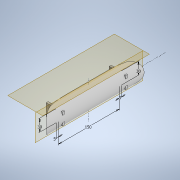
# Autodesk Inventor part: Deckel_Parachute_4
Saved by Autodesk Inventor 2020 (Build 240168000, 168)
## iProperties
Created: 2022-01-25
Part Number: Deckel_Parachute_4
Material: Generisch
Document SubType Name: Modeling
Designer: sp
Density: 1 g/cm^3
Appearance: Vorgabe
Author: sp
## iProperties of the stored document _3D-Druck.ipt
Created: 2022-05-02
Part Number: _3D-Druck
Material: Generisch
Document SubType Name: Modeling
Designer: sp
Density: 1 g/cm^3
Appearance: Vorgabe
Author: sp
Autodesk Inventor part; units mm, degrees
ref_plane "XY Plane" through (0, 0, 0) normal (0, 0, 1) x (1, 0, 0)
sketch "Skizze1" plane through (0, 0, 0) normal (0, 0, 1) x (1, 0, 0)
  circle A0 centre (0, 0) radius 31
  circle A1 centre (0, 0) radius 29
  dimension "d0" = 62
  dimension "d1" = 58
  constraints: 2 centre point, 2 coincident
  measures "d0" diameter of A0
  measures "d1" diameter of A1
extrude "Extrusion1" add sketch "Skizze1" along normal mid plane 300
sketch "Skizze2" plane through (0, 0, 0) normal (0, 1, 0) x (-1, 0, 0)
  line L0 (-11, 169.5773) -> (-11, -169.8146) construction
  line L1 (-74.8376, 0) -> (82.6362, 0) construction
  line L2 (-11, 75) -> (-11, -75)
  line L3 (-31, -150) -> (-31, 150) projected
  line L4 (31, 150) -> (-31, 150) projected
  line L5 (-31, -150) -> (31, -150) projected
  spline S0 degree 2 poles (-11, 75) (-17.8298, 136.4739) (-72.8449, 128.3193) knots 0 0 0 1 1 1
  spline S1 degree 2 poles (-11, -75) (-17.6171, -136.2673) (-74.8376, -130) knots 0 0 0 1 1 1
  line L6 (-72.8449, 128.3193) -> (-74.8376, -130)
  line L7 (-31, 120) -> (-31, 150)
  line L8 (-31, 150) -> (31, 150)
  line L9 (31, 150) -> (31, -150)
  line L10 (31, -150) -> (31, 150) projected
  line L11 (31, -150) -> (-31, -150)
  line L12 (-31, -150) -> (-31, -120)
  point P0 (0, 0)
  dimension "d4" = 11
  dimension "d5" = 150
  dimension "d6" = 30
  dimension "d7" = 30
  constraints: 18 end point, 5 point on line, 3 perpendicular, 2 collinear, 1 horizontal, 1 symmetric about line, 1 vertical, 6 other
  measures "d4" distance from line of point (0, 0) L0
  measures "d5" distance of L2.start L2.end
  measures "d6" distance from line of L7.start L4
  measures "d7" distance from line of L12.end L5
extrude "Extrusion3" cut sketch "Skizze2" along normal mid plane 100 contours S0 L3 L4 L9 L5 S1 L2
ref_plane "Arbeitsebene3" through (0, 33.25, 0) normal (0, 1, 0) x (-1, 0, 0)
sketch "Skizze8" plane through (0, 33.25, 0) normal (0, 1, 0) x (-1, 0, 0)
  line L0 (-11, -75) -> (-11, 75) projected
  arc A0 (-11, 56.4646) -> (-14.2842, 92.4804) centre (-300.1138, 48.2584) ccw
  arc A1 (-11, 56.4646) -> (-14.2842, 92.4804) centre (-31.6354, 72.7405) ccw
  point P0 (0, 0)
  constraints: 4 point on circle, 2 centre point, 1 point on line
extrude "Extrusion6" cut sketch "Skizze8" against normal blind 65
mirror "Spiegeln2" about plane through (0, 0, 0) normal (0, 0, 1) of "Extrusion6"
ref_plane "Arbeitsebene7" through (15, 0, 0) normal (1, 0, 0) x (0, 1, 0)
sketch "Skizze13" plane through (15, 0, 0) normal (1, 0, 0) x (0, 1, 0)
  line L0 (-18, 80) -> (-15, 80)
  line L1 (-15, 80) -> (-15, -80)
  line L2 (-15, -80) -> (-18, -80)
  line L3 (-18, -80) -> (-18, 80)
  line L4 (15, 80) -> (18, 80)
  line L5 (18, 80) -> (18, -80)
  line L6 (18, -80) -> (15, -80)
  line L7 (15, -80) -> (15, 80)
  line L8 (0, 161.0458) -> (0, -181.8657) construction
  line L9 (-78.3289, 0) -> (67.3027, 0) construction
  point P0 (0, 0)
  dimension "d66" = 30
  dimension "d67" = 3
  dimension "d68" = 3
  dimension "d69" = 160
  constraints: 20 end point, 4 parallel, 4 point on line, 3 horizontal, 2 perpendicular, 1 vertical, 2 other
  measures "d66" distance between parallel lines of L7 L1
  measures "d67" distance between parallel lines of L3 L1
  measures "d68" distance between parallel lines of L5 L7
  measures "d69" distance between parallel lines of L2 L0
extrude "Extrusion11" add sketch "Skizze13" against normal mid plane 15
sketch "Skizze14" plane through (15, 0, 0) normal (1, 0, 0) x (0, 1, 0)
  line L0 (-51.8177, 0) -> (40.0312, 0) construction
  line L1 (0, 87.1429) -> (0, -189.8015) construction
  line L2 (-15, 80) -> (15, 80)
  line L3 (15, 80) -> (15, 75)
  line L4 (15, 75) -> (-15, 75)
  line L5 (-15, 75) -> (-15, 80)
  line L6 (-15, -75) -> (15, -75)
  line L7 (15, -75) -> (15, -80)
  line L8 (15, -80) -> (-15, -80)
  line L9 (-15, -80) -> (-15, -75)
  point P0 (0, 0)
  dimension "d72" = 5
  dimension "d73" = 5
  dimension "d74" = 150
  dimension "d75" = 30
  dimension "d76" = 30
  constraints: 20 end point, 4 parallel, 2 horizontal, 2 perpendicular, 2 point on line, 1 vertical, 3 other
  measures "d72" distance of L8.end L6.start
  measures "d73" distance of L4.end L2.start
  measures "d74" distance between parallel lines of L6 L4
  measures "d75" distance of L2.start L2.end
  measures "d76" distance of L7.end L8.end
extrude "Extrusion12" add sketch "Skizze14" against normal blind 25
extrude "Extrusion13" add sketch "Skizze14" along normal blind 15
